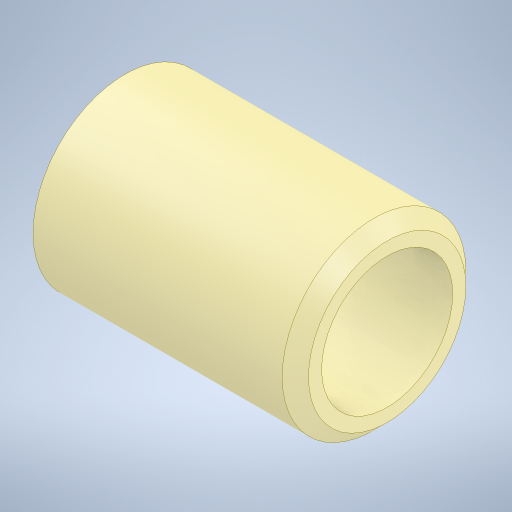
# Autodesk Inventor part: Lager_Schaufelrad
Saved by Autodesk Inventor 2024.4 (Build 284460000, 460)
## iProperties
Created: 2026-01-11
Part Number: Lager_Schaufelrad
Material: Nylon 6/6
Description: Lager_Schaufelrad
Document SubType Name: Modeling
Designer: julia
Mass: 13.4427 g
Surface Area: 65.2678 cm^2
Volume: 11.8962 cm^3
Density: 1.13 g/cm^3
Appearance: Nylon 6
Author: julia
DocNumber: Lager_Schaufelrad.ipt
Folder: I60-Konstruktion\I60-Gruppe-7\Gestell\
VDS_Category: Konstruktion
Masse[kg]: 0,013 kg
Autodesk Inventor part; units mm, degrees
ref_plane "YZ Plane" through (0, 0, 0) normal (1, 0, 0) x (0, 1, 0)
ref_plane "XZ Plane" through (0, 0, 0) normal (0, 1, 0) x (-1, 0, 0)
ref_plane "XY Plane" through (0, 0, 0) normal (0, 0, 1) x (1, 0, 0)
sketch "Skizze1" plane through (0, 0, 0) normal (1, 0, 0) x (0, 1, 0)
  circle A0 centre (0, 0) radius 14
  circle A1 centre (0, 0) radius 10
  dimension "d0" = 28
  dimension "d1" = 20
  constraints: 2 centre point, 2 coincident
  measures "d0" diameter of A0
  measures "d1" diameter of A1
extrude "Extrusion1" add sketch "Skizze1" along normal blind 40
chamfer "Fasen1" distance 2 angle 45 1 edges at (40, -14, 0)
